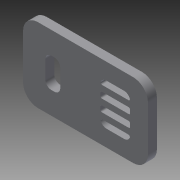
# Autodesk Inventor part: Top Block2
Saved by Autodesk Inventor 2015 (Build 190159000, 159)
## iProperties
Created: 2013-08-06
Part Number: Top Block2
Material: Generic
Document SubType Name: Modeling
Designer: Eric
Density: 1 g/cm^3
Appearance: Default
Author: Eric
Autodesk Inventor part; units mm, degrees
ref_plane "YZ Plane" through (0, 0, 0) normal (1, 0, 0) x (0, 1, 0)
ref_plane "XZ Plane" through (0, 0, 0) normal (0, 1, 0) x (-1, 0, 0)
ref_plane "XY Plane" through (0, 0, 0) normal (0, 0, 1) x (1, 0, 0)
sketch "Sketch1" plane through (0, 0, 0) normal (0, 1, 0) x (-1, 0, 0)
  line L0 (0, -5) -> (32, -5)
  line L1 (32, 20) -> (0, 20)
  line L2 (-5, 15) -> (-5, 0)
  arc A0 (0, 20) -> (-5, 15) centre (0, 15) ccw
  arc A1 (-5, 0) -> (0, -5) centre (0, 0) ccw
  line L3 (3, 0.5) -> (9, 0.5)
  line L4 (9, 14.5) -> (3, 14.5)
  line L5 (1.5858, 12.5) -> (10.4142, 12.5)
  line L6 (1.5, 10.5) -> (10.5, 10.5)
  line L7 (1.5, 8.5) -> (10.5, 8.5)
  line L8 (1.5, 6.5) -> (10.5, 6.5)
  line L9 (1.5, 4.5) -> (10.5, 4.5)
  line L10 (1.5858, 2.5) -> (10.4142, 2.5)
  arc A2 (3, 14.5) -> (1.1144, 13.1667) centre (3, 12.5) ccw
  arc A3 (10.8856, 13.1667) -> (9, 14.5) centre (9, 12.5) ccw
  arc A4 (1.1144, 1.8333) -> (3, 0.5) centre (3, 2.5) ccw
  arc A5 (9, 0.5) -> (10.8856, 1.8333) centre (9, 2.5) ccw
  line L11 (11, 5) -> (11, 6)
  line L12 (1, 6) -> (1, 5)
  line L13 (1, 10) -> (1, 9)
  line L14 (11, 9) -> (11, 10)
  arc A6 (1.5858, 2.5) -> (1.1144, 1.8333) centre (1.5858, 2) ccw
  arc A7 (10.8856, 1.8333) -> (10.4142, 2.5) centre (10.4142, 2) ccw
  arc A8 (10.5, 4.5) -> (11, 5) centre (10.5, 5) ccw
  arc A9 (11, 6) -> (10.5, 6.5) centre (10.5, 6) ccw
  arc A10 (1.5, 6.5) -> (1, 6) centre (1.5, 6) ccw
  arc A11 (1, 5) -> (1.5, 4.5) centre (1.5, 5) ccw
  arc A12 (1, 9) -> (1.5, 8.5) centre (1.5, 9) ccw
  arc A13 (1.5, 10.5) -> (1, 10) centre (1.5, 10) ccw
  arc A14 (11, 10) -> (10.5, 10.5) centre (10.5, 10) ccw
  arc A15 (10.5, 8.5) -> (11, 9) centre (10.5, 9) ccw
  arc A16 (1.1144, 13.1667) -> (1.5858, 12.5) centre (1.5858, 13) ccw
  arc A17 (10.4142, 12.5) -> (10.8856, 13.1667) centre (10.4142, 13) ccw
  arc A18 (37, 15) -> (32, 20) centre (32, 15) ccw
  arc A19 (32, -5) -> (37, 0) centre (32, 0) ccw
  line L15 (37, 15) -> (37, 0)
  line L16 (26.5, 12.5) -> (27.5, 12.5)
  line L17 (29.5, 10.5) -> (29.5, 4.5)
  line L18 (27.5, 2.5) -> (26.5, 2.5)
  line L19 (24.5, 4.5) -> (24.5, 10.5)
  arc A20 (26.5, 12.5) -> (24.5, 10.5) centre (26.5, 10.5) ccw
  arc A21 (29.5, 10.5) -> (27.5, 12.5) centre (27.5, 10.5) ccw
  arc A22 (27.5, 2.5) -> (29.5, 4.5) centre (27.5, 4.5) ccw
  arc A23 (24.5, 4.5) -> (26.5, 2.5) centre (26.5, 4.5) ccw
  point P0 (-5, -5)
  point P1 (-5, 20)
  point P2 (37, -5)
  point P3 (24.5, 12.5)
  point P4 (29.5, 12.5)
  dimension "d0" = 42
  dimension "d2" = 25
  dimension "d3" = 5
  dimension "d4" = 5
  dimension "d5" = 5
  dimension "d8" = 5.5
  dimension "d10" = 2
  dimension "d15" = 2
  dimension "d16" = 2
  dimension "d17" = 2
  dimension "d18" = 2
  dimension "d19" = 2
  dimension "d21" = 2
  dimension "d23" = 0.5
  dimension "d30" = 2
  dimension "d31" = 6
  dimension "d32" = 16
  dimension "d37" = 5
  dimension "d41" = 5
  dimension "d42" = 42
  dimension "d43" = 7.5
  dimension "d44" = 10
  dimension "d45" = 7.5
  dimension "d46" = 2
  dimension "d49" = 5
  constraints: 52 tangent, 48 point on circle, 40 end point, 24 centre point, 18 equal radius, 15 perpendicular, 9 parallel, 9 point on line, 3 horizontal
  measures "d0" distance of point (37, -5) point (-5, -5)
  measures "d2" distance of point (-5, 20) point (-5, -5)
  measures "d3" distance from line of L0 point (0, 0)
  measures "d4" distance from line of point (0, 0) L2
  measures "d5" radius of A0
  measures "d8" distance between parallel lines of L0 L3
  measures "d10" distance between parallel lines of L5 L4
  measures "d15" distance between parallel lines of L7 L6
  measures "d16" distance between parallel lines of L8 L7
  measures "d17" distance between parallel lines of L9 L8
  measures "d18" distance between parallel lines of L10 L9
  measures "d19" radius of A2
  measures "d21" distance between parallel lines of L10 L3
  measures "d23" radius of A6
  measures "d30" distance between parallel lines of L6 L5
  measures "d31" distance between parallel lines of L2 L13
  measures "d32" distance between parallel lines of L2 L14
  measures "d37" radius of A18
  measures "d41" distance of point (24.5, 12.5) point (29.5, 12.5)
  measures "d42" distance between parallel lines of L2 L15
  measures "d43" distance between parallel lines of L15 L17
  measures "d44" distance between parallel lines of L18 L16
  measures "d45" distance between parallel lines of L1 L16
  measures "d46" radius of A20
  measures "d49" radius of A1
extrude "Extrusion2" add sketch "Sketch1" along normal blind 3
body "Solid2"
